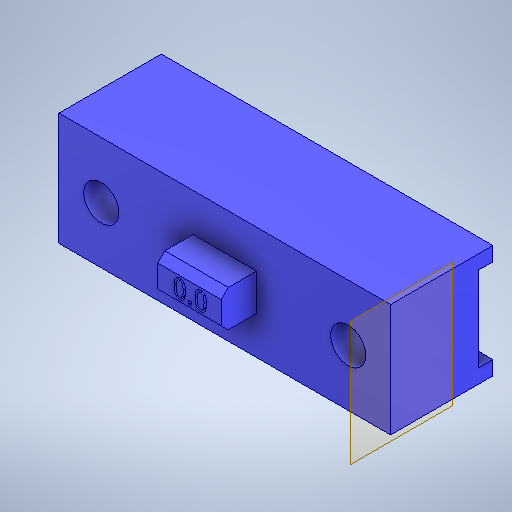
# Autodesk Inventor part: Bearing Spacer_V2_0mm
Saved by Autodesk Inventor 2025.4 (Build 294407000, 407)
## iProperties
Created: 2026-06-01
Part Number: Bearing Spacer_V2_0mm
Material: 일반
Document SubType Name: Modeling
Designer: dalbi
Density: 1 g/cm^3
Appearance: 기본값
Author: dalbi
Autodesk Inventor part; units mm, degrees
ref_plane "YZ Plane" through (0, 0, 0) normal (1, 0, 0) x (0, 1, 0)
ref_plane "XZ Plane" through (0, 0, 0) normal (0, 1, 0) x (-1, 0, 0)
ref_plane "XY Plane" through (0, 0, 0) normal (0, 0, 1) x (1, 0, 0)
ref_plane "작업 평면1" through (23.5, -8, -2) normal (1, 0, 0) x (0, 0, -1)
sketch "스케치1" plane through (23.5, -8, -2) normal (1, 0, 0) x (0, 0, -1)
  line L0 (0, 16) -> (-8.15, 16) projected
  line L1 (-8.15, 16) -> (-8.15, 10.6) projected
  line L2 (-8.15, 10.6) -> (-12.15, 10.6) projected
  line L3 (-13.15, 9.6) -> (-12.15, 10.6) projected
  line L4 (-13.15, 9.6) -> (-13.15, 6.4) projected
  line L5 (-12.15, 5.4) -> (-13.15, 6.4) projected
  line L6 (-12.15, 5.4) -> (-8.15, 5.4) projected
  line L7 (-8.15, 5.4) -> (-8.15, 0) projected
  line L8 (-8.15, 0) -> (0, 0) projected
  line L9 (0, 16) -> (6.35, 16)
  line L10 (6.35, 16) -> (6.35, 15)
  line L11 (4.35, 14) -> (4.35, 2)
  line L12 (4.35, 14) -> (5.35, 14)
  line L13 (0, 0) -> (6.35, 0)
  line L14 (6.35, 0) -> (6.35, 1)
  line L15 (4.35, 2) -> (5.35, 2)
  line L16 (0, 16) -> (-8.15, 16)
  line L17 (-8.15, 10.6) -> (-12.15, 10.6) projected
  line L18 (-8.15, 10.6) -> (-12.15, 10.6)
  line L19 (-12.15, 10.6) -> (-13.15, 9.6)
  line L20 (-13.15, 6.4) -> (-12.15, 5.4)
  line L21 (5.35, 14) -> (6.35, 14)
  line L22 (6.35, 14) -> (6.35, 15)
  line L23 (5.35, 2) -> (6.35, 2)
  line L24 (6.35, 2) -> (6.35, 1)
  point P0 (-2, 8)
  dimension "d1" = 6.35
  constraints: 30 end point, 5 horizontal, 4 perpendicular, 2 collinear, 1 vertical
  measures "d1" distance of L0.start L9.end
sketch "스케치2" plane through (-23.5, 8, 6.15) normal (0, 0, 1) x (1, 0, 0)
  arc A0 (7.9209, -9.6) -> (7.9209, -6.4) centre (6, -8) ccw projected
  line L0 (39.0791, -9.6) -> (7.9209, -9.6) projected
  circle A1 centre (6, -8) radius 2.5
  circle A2 centre (41, -8) radius 2.5 projected
  circle A3 centre (41, -8) radius 2.5
  point P0 (23.5, -8)
  point P1 (7.9209, -6.4)
  constraints: 2 coincident, 1 centre point, 4 other
extrude "돌출1" add sketch "스케치1" against normal up to surface (47 mm away)
extrude "돌출2" cut sketch "스케치2" along normal mid plane 50
sketch "스케치3" plane through (-15.5791, 1.6, 11.15) normal (0, 0, 1) x (1, 0, 0)
  line L0 (15.5791, -14.4593) -> (15.5791, 15.5737)
  line L1 (-7.9209, 4.4) -> (-7.9209, -7.6) projected
  line L2 (-7.9209, 4.4) -> (11.0791, 4.4)
  line L3 (11.0791, 4.4) -> (11.0791, -7.6)
  line L4 (11.0791, -7.6) -> (-7.9209, -7.6)
  line L5 (-7.9209, -7.6) -> (-7.9209, 4.4)
  line L6 (39.0791, 4.4) -> (39.0791, -7.6)
  line L7 (39.0791, 4.4) -> (20.0791, 4.4)
  line L8 (20.0791, 4.4) -> (20.0791, -7.6)
  line L9 (20.0791, -7.6) -> (39.0791, -7.6)
  line L10 (39.0791, -7.6) -> (39.0791, 4.4)
  point P0 (15.5791, -1.6)
  dimension "d9" = 19
  constraints: 20 end point, 5 symmetric about line, 2 parallel, 1 horizontal, 1 perpendicular, 1 vertical
  measures "d9" distance of L1.start L2.end
extrude "돌출3" cut sketch "스케치3" against normal up to surface (5 mm away)
sketch "스케치4" plane through (-4.5, 1.6, 11.15) normal (0, 0, 1) x (1, 0, 0)
  line L0 (2.1691, -0.2851) -> (8.7999, -0.2851) construction
  line L1 (8.7999, -0.2851) -> (8.7999, -2.6545) construction
  line L2 (8.7999, -2.6545) -> (2.1691, -2.6545) construction
  line L3 (2.1691, -2.6545) -> (2.1691, -0.2851) construction
  spline S0 degree 2 poles (3.9352, -1.6066) (3.9352, -2.29) (3.5379, -2.9301) (3.1242, -2.9301) knots 0 0 0 1 2 2 2
  spline S1 degree 2 poles (3.1242, -2.9301) (2.7043, -2.9301) (2.3111, -2.2776) (2.3111, -1.6087) knots 0 0 0 1 2 2 2
  spline S2 degree 2 poles (2.3111, -1.6087) (2.3111, -0.9212) (2.7084, -0.2851) (3.1242, -0.2851) knots 0 0 0 1 2 2 2
  spline S3 degree 2 poles (3.1242, -0.2851) (3.542, -0.2851) (3.9352, -0.9438) (3.9352, -1.6066) knots 0 0 0 1 2 2 2
  spline S4 degree 2 poles (3.4988, -2.3805) (3.5482, -2.255) (3.5894, -1.868) (3.5894, -1.6066) knots 0 0 0 1 2 2 2
  spline S5 degree 2 poles (3.5894, -1.6066) (3.5894, -1.3452) (3.5482, -0.9603) (3.4967, -0.8306) knots 0 0 0 1 2 2 2
  spline S6 degree 2 poles (3.4967, -0.8306) (3.4453, -0.7009) (3.2662, -0.5671) (3.1242, -0.5671) knots 0 0 0 1 2 2 2
  spline S7 degree 2 poles (3.1242, -0.5671) (2.9822, -0.5671) (2.799, -0.7009) (2.7454, -0.8347) knots 0 0 0 1 2 2 2
  spline S8 degree 2 poles (2.7454, -0.8347) (2.694, -0.9644) (2.6569, -1.3596) (2.6569, -1.6087) knots 0 0 0 1 2 2 2
  spline S9 degree 2 poles (2.6569, -1.6087) (2.6569, -1.8762) (2.6899, -2.2344) (2.7434, -2.3744) knots 0 0 0 1 2 2 2
  spline S10 degree 2 poles (2.7434, -2.3744) (2.7928, -2.5061) (2.976, -2.6481) (3.1242, -2.6481) knots 0 0 0 1 2 2 2
  spline S11 degree 2 poles (3.1242, -2.6481) (3.2641, -2.6481) (3.4473, -2.5143) (3.4988, -2.3805) knots 0 0 0 1 2 2 2
  line L4 (4.8058, -2.8766) -> (4.3983, -2.8766)
  line L5 (4.3983, -2.8766) -> (4.3983, -2.3908)
  line L6 (4.3983, -2.3908) -> (4.8058, -2.3908)
  line L7 (4.8058, -2.3908) -> (4.8058, -2.8766)
  spline S12 degree 2 poles (6.8992, -1.6066) (6.8992, -2.29) (6.5019, -2.9301) (6.0882, -2.9301) knots 0 0 0 1 2 2 2
  spline S13 degree 2 poles (6.0882, -2.9301) (5.6683, -2.9301) (5.2752, -2.2776) (5.2752, -1.6087) knots 0 0 0 1 2 2 2
  spline S14 degree 2 poles (5.2752, -1.6087) (5.2752, -0.9212) (5.6724, -0.2851) (6.0882, -0.2851) knots 0 0 0 1 2 2 2
  spline S15 degree 2 poles (6.0882, -0.2851) (6.506, -0.2851) (6.8992, -0.9438) (6.8992, -1.6066) knots 0 0 0 1 2 2 2
  spline S16 degree 2 poles (6.4628, -2.3805) (6.5122, -2.255) (6.5534, -1.868) (6.5534, -1.6066) knots 0 0 0 1 2 2 2
  spline S17 degree 2 poles (6.5534, -1.6066) (6.5534, -1.3452) (6.5122, -0.9603) (6.4608, -0.8306) knots 0 0 0 1 2 2 2
  spline S18 degree 2 poles (6.4608, -0.8306) (6.4093, -0.7009) (6.2302, -0.5671) (6.0882, -0.5671) knots 0 0 0 1 2 2 2
  spline S19 degree 2 poles (6.0882, -0.5671) (5.9462, -0.5671) (5.763, -0.7009) (5.7095, -0.8347) knots 0 0 0 1 2 2 2
  spline S20 degree 2 poles (5.7095, -0.8347) (5.658, -0.9644) (5.621, -1.3596) (5.621, -1.6087) knots 0 0 0 1 2 2 2
  spline S21 degree 2 poles (5.621, -1.6087) (5.621, -1.8762) (5.6539, -2.2344) (5.7074, -2.3744) knots 0 0 0 1 2 2 2
  spline S22 degree 2 poles (5.7074, -2.3744) (5.7568, -2.5061) (5.94, -2.6481) (6.0882, -2.6481) knots 0 0 0 1 2 2 2
  spline S23 degree 2 poles (6.0882, -2.6481) (6.2282, -2.6481) (6.4114, -2.5143) (6.4628, -2.3805) knots 0 0 0 1 2 2 2
  point P0 (4.5, -1.6)
  constraints: 2 other
extrude "돌출4" cut sketch "스케치4" against normal blind 5
